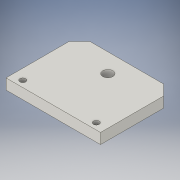
# Autodesk Inventor part: Werkstück_C
Saved by Autodesk Inventor 2018.3 (Build 223284000, 284)
## iProperties
RuleStatus: InUse
Created: 2019-11-28
Material: Stahl, unlegiert
Document SubType Name: Modeling
Designer: dirkb
Density: 7.85 g/cm^3
Appearance: Stahl
Description: Werkstück
Part Number: Werkstück_C
Werkstoff: S235JRC+C
Author: dirkb
Autodesk Inventor part; units mm, degrees
ref_plane "YZ Plane" through (0, 0, 0) normal (1, 0, 0) x (0, 1, 0)
ref_plane "XZ Plane" through (0, 0, 0) normal (0, 1, 0) x (-1, 0, 0)
ref_plane "XY Plane" through (0, 0, 0) normal (0, 0, 1) x (1, 0, 0)
sketch "Skizze_Grundkörper" plane through (0, 0, 0) normal (0, 0, 1) x (1, 0, 0)
  line L0 (-63, 0) -> (63, 0) projected
  line L1 (0, -49) -> (0, 49) projected
  line L2 (45, -35) -> (-45, -35)
  line L3 (-45, -35) -> (-45, 35)
  line L4 (-45, 35) -> (45, 35)
  line L5 (45, 35) -> (45, -35)
  line L6 (45, -35) -> (-45, 35) construction
  line L7 (-45, -35) -> (45, 35) construction
  point P0 (0, 0)
  dimension "Länge" = 90
  dimension "Höhe" = 70
  constraints: 12 end point, 2 midpoint, 2 parallel, 1 horizontal, 1 perpendicular
  measures "Länge" distance of L3.end L4.end
  measures "Höhe" distance of L4.end L2.start
extrude "Grundkörper" add sketch "Skizze_Grundkörper" along normal blind 10
sketch "Skizze2" plane through (0, 0, 10) normal (0, 0, 1) x (1, 0, 0)
  line L0 (-45, -35) -> (45, -35) projected
  line L1 (45, -35) -> (45, 35) projected
  line L2 (45, 35) -> (-45, 35) projected
  line L3 (-45, 35) -> (-45, -35) projected
  line L4 (-63, 0) -> (63, 0) projected
  line L5 (0, -49) -> (0, 49) projected
  point P0 (0, 0)
  point P1 (0, 17)
  dimension "d4" = 52
  constraints: 1 point on line
  measures "d4" distance from line of L0 point (0, 17)
hole "Bohrung_9,7_mm" at (0, 17, 10) direction (0, 0, -1) diameter 9.7 end through all
sketch "Skizze3" plane through (0, 0, 10) normal (0, 0, 1) x (1, 0, 0)
  circle A0 centre (0, 17) radius 4.85 projected
  line L0 (-45, -35) -> (45, -35) projected
  line L1 (45, -35) -> (45, 35) projected
  line L2 (45, 35) -> (-45, 35) projected
  line L3 (-45, 35) -> (-45, -35) projected
  line L4 (-63, 0) -> (63, 0) projected
  line L5 (0, -49) -> (0, 49) projected
  point P0 (0, 0)
  point P1 (-35, -29)
  point P2 (35, -29)
  dimension "d12" = 70
  dimension "d13" = 6
  constraints: 1 symmetric about line
  measures "d12" distance of point (35, -29) point (-35, -29)
  measures "d13" distance from line of L0 point (35, -29)
hole "Bohrung_5,5_mm" at (-35, -29, 10) at (35, -29, 10) direction (0, 0, -1) diameter 5.5 end through all
chamfer "Fase_10_mm" distance 10 angle 45 2 edges at (-45, 35, 5) (45, 35, 5)
